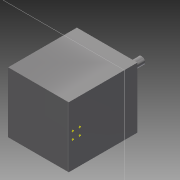
# Autodesk Inventor part: NEMA_17
Saved by Autodesk Inventor 2013 (Build 170138000, 138)
## iProperties
Created: 2013-09-16
Part Number: NEMA_17
Material: Steel, Carbon
Document SubType Name: Modeling
Designer: Ian
Density: 7.87 g/cm^3
Mass: 684.632 g
Surface Area: 123.23 cm^2
Volume: 86.9927 cm^3
GlobalPropertyList: <PropertyList/>
Author: Ian
Autodesk Inventor part; units mm, degrees
ref_plane "YZ Plane" through (0, 0, 0) normal (1, 0, 0) x (0, 1, 0)
ref_plane "XZ Plane" through (0, 0, 0) normal (0, 1, 0) x (-1, 0, 0)
ref_plane "XY Plane" through (0, 0, 0) normal (0, 0, 1) x (1, 0, 0)
sketch "Sketch1" plane through (0, 0, 0) normal (0, 1, 0) x (-1, 0, 0)
  line L0 (-21.15, -21.15) -> (21.15, -21.15)
  line L1 (21.15, -21.15) -> (21.15, 21.15)
  line L2 (21.15, 21.15) -> (-21.15, 21.15)
  line L3 (-21.15, 21.15) -> (-21.15, -21.15)
  line L4 (-21.15, -21.15) -> (21.15, 21.15) construction
  line L5 (21.15, -21.15) -> (-21.15, 21.15) construction
  point P0 (0, 0)
  dimension "d0" = 42.3
  dimension "d1" = 42.3
  constraints: 12 end point, 2 midpoint, 2 parallel, 1 horizontal, 1 perpendicular
  measures "d0" distance of L2.end L1.end
  measures "d1" distance of L1.end L0.end
extrude "Extrusion1" add sketch "Sketch1" along normal blind 48
sketch "Sketch2" plane through (0, 48, 0) normal (0, 1, 0) x (1, 0, 0)
  circle A0 centre (0, 0) radius 11
  dimension "d4" = 22
  constraints: 1 centre point, 1 coincident
  measures "d4" diameter of A0
extrude "Extrusion2" add sketch "Sketch2" along normal blind 2
sketch "Sketch3" plane through (0, 50, 0) normal (0, 1, 0) x (1, 0, 0)
  circle A0 centre (0, 0) radius 11 projected
  circle A1 centre (0, 0) radius 2.5
  dimension "d7" = 5
  constraints: 1 centre point, 1 coincident
  measures "d7" diameter of A1
extrude "Extrusion3" add sketch "Sketch3" along normal blind 22 contours A1
sketch "Sketch4" plane through (0, 48, 0) normal (0, 1, 0) x (1, 0, 0)
  circle A0 centre (0, 0) radius 11 projected
  line L0 (-15.5, 15.5) -> (15.5, 15.5) construction
  line L1 (15.5, 15.5) -> (15.5, -15.5) construction
  line L2 (15.5, -15.5) -> (-15.5, -15.5) construction
  line L3 (-15.5, -15.5) -> (-15.5, 15.5) construction
  dimension "d10" = 31
  dimension "d11" = 31
  dimension "d12" = 15.5
  dimension "d13" = 15.5
  constraints: 8 end point, 4 coincident, 2 parallel, 1 horizontal, 1 perpendicular
  measures "d10" distance of L1.end L2.end
  measures "d11" distance of L0.end L1.end
  measures "d12" distance from line of L0 A0.centre
  measures "d13" distance from line of L1 A0.centre
hole "Hole1" at (-15.5, 48, -15.5) at (15.5, 48, -15.5) at (15.5, 48, 15.5) at (-15.5, 48, 15.5) direction (0, -1, 0) diameter 2.459 depth 4.5 thread size "M3x0.5" class "6H" standard "ISO Metric profile"
sketch "Sketch5" plane through (21.15, 0, 21.15) normal (1, 0, 0) x (0, 0, -1)
  line L0 (0, 0) -> (42.3, 0) projected
  line L1 (42.3, 0) -> (42.3, 48) projected
  line L2 (0, 48) -> (42.3, 48) projected
  line L3 (0, 0) -> (0, 48) projected
  line L4 (26.15, 0) -> (26.15, 10)
  line L5 (26.15, 10) -> (16.15, 10)
  line L6 (16.15, 10) -> (16.15, 0)
  line L7 (16.15, 10) -> (26.15, 0)
  line L8 (26.15, 10) -> (16.15, 0)
  line L9 (18.65, 2.5) -> (23.65, 2.5)
  line L10 (23.65, 2.5) -> (23.65, 7.5)
  line L11 (23.65, 7.5) -> (18.65, 7.5)
  line L12 (18.65, 7.5) -> (18.65, 2.5)
  line L13 (18.65, 2.5) -> (23.65, 7.5) construction
  line L14 (23.65, 2.5) -> (18.65, 7.5) construction
  point P0 (21.15, 0)
  point P1 (21.15, 5)
  dimension "d23" = 16.15
  dimension "d24" = 16.15
  dimension "d26" = 10
  dimension "d27" = 10
  dimension "d28" = 5
  dimension "d29" = 5
  constraints: 22 end point, 4 coincident, 3 midpoint, 3 parallel, 2 point on line, 1 horizontal, 1 perpendicular
  measures "d23" distance between parallel lines of L1 L4
  measures "d24" distance between parallel lines of L3 L6
  measures "d26" distance of L5.end L6.end
  measures "d27" distance of L4.start L4.end
  measures "d28" distance of L11.end L10.end
  measures "d29" distance of L10.end L9.end
body "Solid1"
